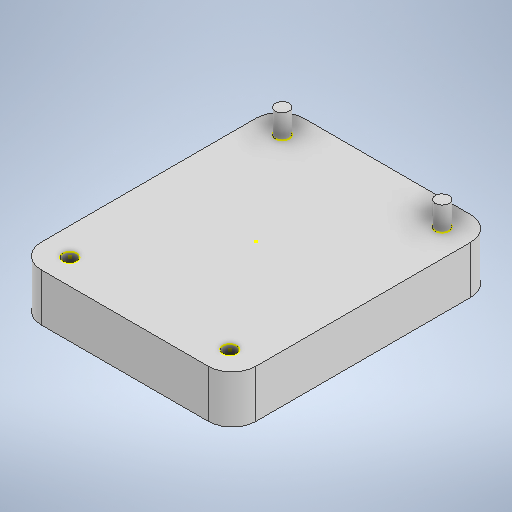
# Autodesk Inventor part: BASE RELE
Saved by Autodesk Inventor 2025 (Build 290162000, 162)
## iProperties
Created: 2024-09-28
Part Number: BASE RELE
Material: Genérico
Document SubType Name: Modeling
Designer: phmca
Density: 1 g/cm^3
Appearance: Padrão
Author: phmca
Autodesk Inventor part; units mm, degrees
ref_plane "YZ Plane" through (0, 0, 0) normal (1, 0, 0) x (0, 1, 0)
ref_plane "XZ Plane" through (0, 0, 0) normal (0, 1, 0) x (-1, 0, 0)
ref_plane "XY Plane" through (0, 0, 0) normal (0, 0, 1) x (1, 0, 0)
sketch "Esboço1" plane through (0, 0, 0) normal (0, 1, 0) x (-1, 0, 0)
  line L0 (-22.5, 27.5) -> (22.5, 27.5)
  line L1 (22.5, 27.5) -> (22.5, -27.5)
  line L2 (22.5, -27.5) -> (-22.5, -27.5)
  line L3 (-22.5, -27.5) -> (-22.5, 27.5)
  line L4 (-22.5, 27.5) -> (22.5, -27.5) construction
  line L5 (22.5, 27.5) -> (-22.5, -27.5) construction
  circle A0 centre (16.75, -22.25) radius 1.45
  circle A1 centre (16.75, 22.25) radius 1.45
  circle A2 centre (-16.75, 22.25) radius 1.45
  circle A3 centre (-16.75, -22.25) radius 1.45
  line L6 (-16.75, 22.25) -> (-16.75, -22.25) construction
  line L7 (-16.75, -22.25) -> (16.75, -22.25) construction
  line L8 (16.75, -22.25) -> (16.75, 22.25) construction
  line L9 (16.75, 22.25) -> (-16.75, 22.25) construction
  line L10 (0, 0) -> (9.1939, 0)
  line L11 (0, 0) -> (0, -6.5379)
  line L12 (16.75, 0) -> (30.08, 0) construction
  line L13 (0, 22.25) -> (0, 28.3312) construction
  dimension "d0" = 2.9
  dimension "d1" = 2.9
  dimension "d2" = 2.9
  dimension "d3" = 2.9
  dimension "d4" = 33.5
  dimension "d5" = 44.5
  dimension "d6" = 55
  dimension "d7" = 45
  constraints: 28 end point, 4 centre point, 4 horizontal, 4 midpoint, 3 perpendicular, 3 vertical, 2 collinear, 2 parallel
  measures "d0" diameter of A0
  measures "d1" diameter of A1
  measures "d2" diameter of A2
  measures "d3" diameter of A3
  measures "d4" distance of L6.end L7.end
  measures "d5" distance of L7.end L8.end
  measures "d6" distance of L0.end L1.end
  measures "d7" distance between parallel lines of L3 L1
extrude "Extrusão1" add sketch "Esboço1" along normal blind 10 contours L0 L1 L2 L3 | A0 | A1 | A2 | A3
sketch "Esboço2" plane through (0, 10, 0) normal (0, 1, 0) x (1, 0, 0)
  circle A0 centre (16.75, -22.25) radius 1.45 projected
  circle A1 centre (-16.75, -22.25) radius 1.45 projected
  circle A2 centre (16.75, 22.25) radius 1.45 projected
  circle A3 centre (-16.75, 22.25) radius 1.45 projected
  point P0 (0, 0)
extrude "Extrusão2" cut sketch "Esboço2" against normal blind 8.5 contours A0 | A1
extrude "Extrusão3" add sketch "Esboço2" along normal blind 5 contours A2 | A3
fillet "Arredondamento1" radius 5 4 edges at (22.5, 5, 27.5) (22.5, 5, -27.5) (-22.5, 5, -27.5) (-22.5, 5, 27.5)
